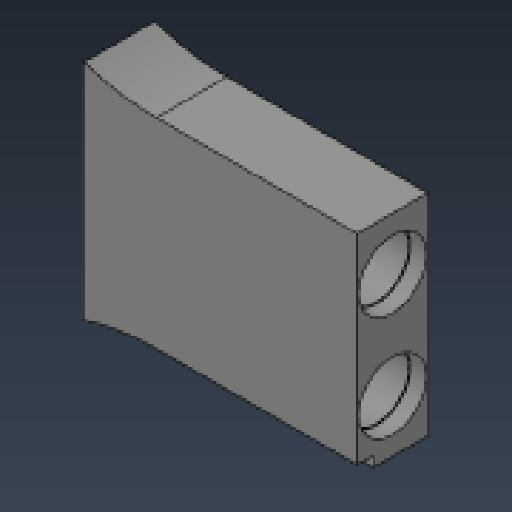
# Autodesk Inventor part: BearigHold
Saved by Autodesk Inventor 2026.2 (Build 302298010, 298A)
## iProperties
Created: 2026-04-04
Part Number: BearigHold
Material: Generic
Document SubType Name: Modeling
Designer: szymo
Density: 1 g/cm^3
Appearance: Default(1)
Author: szymo
Autodesk Inventor part; units mm, degrees
ref_plane "YZ Plane" through (0, 0, 0) normal (1, 0, 0) x (0, 1, 0)
ref_plane "XZ Plane" through (0, 0, 0) normal (0, 1, 0) x (-1, 0, 0)
ref_plane "XY Plane" through (0, 0, 0) normal (0, 0, 1) x (1, 0, 0)
ref_plane "Work Plane1" through (11.7, -32.6479, 0) normal (0, 0, 1) x (-1, 0, 0)
sketch "Sketch1" plane through (11.7, -32.6479, 0) normal (0, 0, 1) x (-1, 0, 0)
  circle A0 centre (14.5, -14.5) radius 13.85 projected
  circle A1 centre (14.5, -14.5) radius 14.5 projected
  circle A2 centre (14.5, -55.2958) radius 13.85 projected
  circle A3 centre (14.5, -55.2958) radius 14.5 projected
  circle A4 centre (13, -35.0012) radius 5 projected
  line L0 (0, 0) -> (33.1738, 0)
  line L1 (33.1738, 0) -> (33.1738, -67)
  line L2 (33.1738, -67) -> (0, -67)
  line L3 (0, -67) -> (0, 0)
  line L4 (2, 0) -> (2, -67)
  line L5 (14.5, -28.35) -> (2, -28.35)
  line L6 (14.5, -29) -> (2, -29)
  line L7 (14.5, -40.7958) -> (2, -40.7958)
  line L8 (14.5, -41.4458) -> (2, -41.4458)
  line L9 (19, 0) -> (19, -67)
  point P0 (11.7, -32.6479)
  point P1 (19, -42.1973)
  point P2 (19, -27.5986)
  point P3 (19, -41.5118)
  point P4 (19, -28.284)
  dimension "d0" = 67
  dimension "d1" = 2
  dimension "d2" = 1
  constraints: 20 end point, 8 point on line, 7 perpendicular, 5 horizontal, 2 parallel, 1 coincident, 9 other
  measures "d0" distance of L2.end L0.start
  measures "d1" distance between parallel lines of L4 L3
  measures "d2" distance edge to line of A4 L9
ref_plane "Work Plane2" through (-23.2799, 2.168, 4) normal (0, 0, -1) x (-0.6704745, 0.7419326, 0)
ref_plane "Work Plane4" through (-17.5791, -32.927, 4.9) normal (0, 0, -1) x (0.0194385, 0.9998111, 0)
ref_plane "Work Plane7" through (-17.5791, -32.927, 3.4) normal (0, 0, -1) x (0.0194385, 0.9998111, 0)
extrude "Extrusion1" add sketch "Sketch1" along normal up to surface (3.4 mm away) contours L9 A1 L5 A0 | L9 A3 L7 L4 L6 A1 | A1 L6 L4 L5 | L9 A2 L8 A3 | A3 L8 L4 L7
ref_plane "Work Plane3" through (-21.8144, -37.1623, 4.9) normal (0, 0, -1) x (-0.3909035, 0.9204317, 0)
ref_plane "Work Plane5" through (-22.6017, 2.8462, 5.5) normal (0, 0, -1) x (0.4990785, 0.8665568, 0)
ref_plane "Work Plane8" through (-22.6017, 2.8462, 4) normal (0, 0, -1) x (0.4990785, 0.8665568, 0)
extrude "Extrusion2" add sketch "Sketch1" along normal up to surface (4 mm away) contours L9 A3 L7 L4 L6 A1 | L9 A2 L8 A3 | A3 L8 L4 L7
ref_plane "Work Plane6" through (11.7, -32.6479, 5.3) normal (0, 0, 1) x (1, 0, 0)
sketch "Sketch2" plane through (11.7, -32.6479, 4) normal (0, 0, 1) x (1, 0, 0)
  circle A0 centre (-13, 35.0012) radius 5 projected
  line L0 (-2, 41.4458) -> (-14.5, 41.4458) projected
  arc A1 (-19, 42.1973) -> (-14.5, 41.4458) centre (-14.5, 55.2958) ccw projected
  line L1 (-19, 42.1973) -> (-19, 28.284) projected
  arc A2 (-14.5, 29) -> (-19, 28.284) centre (-14.5, 14.5) ccw projected
  line L2 (-14.5, 29) -> (-2, 29) projected
  line L3 (-2, 29) -> (-2, 41.4458) projected
  point P0 (-11.7, 32.6479)
extrude "Extrusion4" add sketch "Sketch2" along normal blind 0.4 and the other way blind 0.2 contours A0 | L3 L2 A2 L1 A1 L0
sketch "Sketch3" plane through (9.7, -4.2979, 0) normal (1, 0, 0) x (0, 0, -1)
  line L0 (0, 0) -> (-3.4, 0) projected
  line L1 (0, 0) -> (0, 13.0958) projected
  line L2 (0, 13.0958) -> (-4.4, 13.0958) projected
  line L3 (-4.4, 6.5479) -> (0, 6.5479)
  line L4 (-4.4, 6.5479) -> (0, 0)
  line L5 (-4.4, 6.5479) -> (0, 13.0958)
  line L6 (0, 6.5479) -> (-2.2, 9.8219)
  line L7 (0, 6.5479) -> (-2.2, 3.274)
  line L8 (-3.4, 0.65) -> (-4.4, 0.65) projected
  line L9 (-3.4, 0) -> (-3.4, 0.65) projected
  line L10 (-4.4, 0.65) -> (-4.4, 13.0958) projected
  line L11 (-4.4, 0.65) -> (-4.4, 13.0958) projected
  point P0 (0, 4.2979)
  dimension "d11" = 6.5479
  dimension "d12" = 6.5479
  constraints: 10 end point, 3 midpoint, 2 coincident, 1 perpendicular, 1 point on line
  measures "d11" distance between parallel lines of L0 L3
  measures "d12" distance between parallel lines of L2 L3
hole "Hole1" at (9.7, -1.024, 2.2) at (9.7, 5.524, 2.2) direction (-1, 0, 0) diameter 4 depth 5.5 counterbore diameter 4.2 counterbore depth 1
equation "\"d11\" = d12"
body "Solid1"
